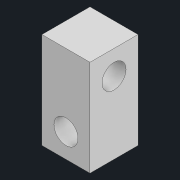
# Autodesk Inventor part: UnionOrtogonal
Saved by Autodesk Inventor 2021 (Build 250183000, 183)
## iProperties
Created: 2021-05-06
Part Number: UnionOrtogonal
Material: Generic
Document SubType Name: Modeling
Designer: GABRIEL LOL
Density: 1 g/cm^3
Appearance: Default
Author: GABRIEL LOL
Autodesk Inventor part; units mm, degrees
ref_plane "YZ Plane" through (0, 0, 0) normal (1, 0, 0) x (0, 1, 0)
ref_plane "XZ Plane" through (0, 0, 0) normal (0, 1, 0) x (-1, 0, 0)
ref_plane "XY Plane" through (0, 0, 0) normal (0, 0, 1) x (1, 0, 0)
sketch "Sketch1" plane through (0, 0, 0) normal (0, 0, 1) x (1, 0, 0)
  circle A0 centre (0, 0) radius 1.25
  line L0 (0, 0) -> (0, 5) construction
  circle A1 centre (0, 5) radius 1.25 construction
  line L1 (0, 0) -> (-2.5, 0) construction
  line L2 (-2.5, 0) -> (-2.5, -2.5) construction
  line L3 (0, 5) -> (0, 7.5) construction
  line L4 (0, 7.5) -> (2.5, 7.5) construction
  line L5 (-2.5, -2.5) -> (2.5, -2.5)
  line L6 (2.5, -2.5) -> (2.5, 7.5)
  line L7 (2.5, 7.5) -> (-2.5, 7.5)
  line L8 (-2.5, 7.5) -> (-2.5, -2.5)
  dimension "d0" = 2.5
  dimension "d1" = 5
  dimension "d2" = 2.5
  dimension "d3" = 2.5
  dimension "d4" = 2.5
  dimension "d5" = 2.5
  dimension "d6" = 2.5
  constraints: 18 end point, 3 perpendicular, 2 centre point, 2 coincident, 2 horizontal, 2 parallel, 2 vertical
  measures "d0" diameter of A0
  measures "d1" distance of L0.start L0.end
  measures "d2" diameter of A1
  measures "d3" distance of L0.start L1.end
  measures "d4" distance of L1.end L2.end
  measures "d5" distance of L3.start L3.end
  measures "d6" distance of L3.end L4.end
extrude "Extrusion1" add sketch "Sketch1" along normal blind 5
sketch "Sketch2" plane through (2.5, -2.5, 0) normal (1, 0, 0) x (0, 0, -1)
  line L0 (-5, 1.25) -> (-5, 3.75) projected
  line L1 (0, 0) -> (0, 10) projected
  line L2 (0, 10) -> (-5, 10) projected
  line L3 (-5, 0) -> (-5, 10) projected
  line L4 (0, 0) -> (-5, 0) projected
  line L5 (-5, 0) -> (-5, 10) construction
  line L6 (-5, 2.5) -> (-2.5, 2.5) construction
  line L7 (-2.5, 2.5) -> (-2.5, 2.5) construction
  line L8 (-2.5, 2.5) -> (-2.5, 7.5) construction
  circle A0 centre (-2.5, 7.5) radius 1.25
  point P0 (0, 2.5)
  dimension "d9" = 2.5
  dimension "d10" = 0
  dimension "d11" = 5
  dimension "d12" = 2.5
  constraints: 6 end point, 2 perpendicular, 2 point on line, 1 centre point, 1 coincident
  measures "d9" distance of L6.start L6.end
  measures "d10" distance of L6.end L7.end
  measures "d11" distance of L7.end L8.end
  measures "d12" diameter of A0
extrude "Extrusion2" cut sketch "Sketch2" against normal blind 5 contours A0
body "Solid1"
